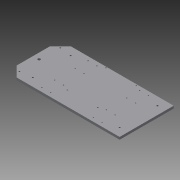
# Autodesk Inventor part: BaseNEW
Saved by Autodesk Inventor 2015 (Build 190159000, 159)
## iProperties
Created: 2015-04-03
Part Number: BaseNEW
Material: Generic
Document SubType Name: Modeling
Designer: Judson
Density: 1 g/cm^3
Appearance: Default
Author: Judson
Autodesk Inventor part; units mm, degrees
ref_plane "YZ Plane" through (0, 0, 0) normal (1, 0, 0) x (0, 1, 0)
ref_plane "XZ Plane" through (0, 0, 0) normal (0, 1, 0) x (-1, 0, 0)
ref_plane "XY Plane" through (0, 0, 0) normal (0, 0, 1) x (1, 0, 0)
sketch "Sketch1" plane through (0, 0, 0) normal (0, 1, 0) x (-1, 0, 0)
  line L0 (139.7, 66.675) -> (-139.7, 66.675)
  line L1 (-139.7, 66.675) -> (-139.7, -66.675)
  line L2 (-139.7, -66.675) -> (139.7, -66.675)
  line L3 (139.7, -66.675) -> (139.7, 66.675)
  line L4 (114.3, 66.675) -> (114.3, -66.675)
  line L5 (114.3, 66.675) -> (139.7, 41.275)
  line L6 (114.3, -66.675) -> (139.7, -41.275)
  point P0 (0, 0)
  dimension "d0" = 133.35
  dimension "d1" = 279.4
  dimension "d2" = 66.675
  dimension "d3" = 139.7
  dimension "d4" = 25.4
  dimension "d5" = 45
  dimension "d6" = 45
  constraints: 14 end point, 4 point on line, 2 parallel, 2 perpendicular, 1 horizontal
  measures "d0" distance of L0.end L1.end
  measures "d1" distance of L1.end L2.end
  measures "d2" distance from line of point (0, 0) L2
  measures "d3" distance from line of point (0, 0) L1
  measures "d4" distance between parallel lines of L4 L3
  measures "d5" angle of L2 L6
  measures "d6" angle of L4 L5
extrude "Body" add sketch "Sketch1" along normal blind 5.9944 contours L4 L2 L1 L0 | L5 L3 L6 L4
sketch "Sketch2" plane through (0, 5.9944, 0) normal (0, 1, 0) x (1, 0, 0)
  line L0 (-114.3, 66.675) -> (-139.7, 41.275) projected
  line L1 (-139.7, 41.275) -> (-139.7, -41.275) projected
  line L2 (-139.7, -41.275) -> (-114.3, -66.675) projected
  line L3 (-114.3, -66.675) -> (139.7, -66.675) projected
  line L4 (139.7, -66.675) -> (139.7, 66.675) projected
  line L5 (139.7, 66.675) -> (-114.3, 66.675) projected
  line L6 (-114.3, -66.675) -> (-114.3, 66.675)
  line L7 (-114.3, -14.605) -> (139.7, -14.605)
  line L8 (76.2, -14.605) -> (76.2, -66.675)
  line L9 (-50.8, -14.605) -> (-50.8, -66.675)
  line L10 (-114.3, -66.675) -> (139.7, -66.675) projected
  line L11 (-40.005, -14.605) -> (-40.005, -66.675)
  line L12 (-40.005, -66.675) -> (-61.595, -66.675)
  line L13 (-61.595, -66.675) -> (-61.595, -14.605)
  line L14 (12.7, -66.675) -> (12.7, 66.675)
  line L15 (76.2, -14.605) -> (76.2, -66.675)
  line L16 (65.405, -14.605) -> (65.405, -66.675)
  line L17 (86.995, -66.675) -> (86.995, -14.605)
  circle A0 centre (-61.595, -57.023) radius 1.27
  circle A1 centre (-61.595, -25.273) radius 1.27
  circle A2 centre (-40.005, -57.023) radius 1.27
  circle A3 centre (-40.005, -25.273) radius 1.27
  circle A4 centre (86.995, -57.023) radius 1.27
  circle A5 centre (86.995, -25.273) radius 1.27
  circle A6 centre (65.405, -25.273) radius 1.27
  circle A7 centre (65.405, -57.023) radius 1.27
  line L18 (-139.7, 0) -> (139.7, 0)
  line L19 (-114.3, 14.605) -> (139.7, 14.605)
  line L20 (76.2, 14.605) -> (76.2, 66.675)
  line L21 (-50.8, 14.605) -> (-50.8, 66.675)
  line L22 (-40.005, 14.605) -> (-40.005, 66.675)
  line L23 (-61.595, 66.675) -> (-61.595, 14.605)
  line L24 (65.405, 14.605) -> (65.405, 66.675)
  line L25 (86.995, 66.675) -> (86.995, 14.605)
  circle A8 centre (-61.595, 57.023) radius 1.27
  circle A9 centre (-61.595, 25.273) radius 1.27
  circle A10 centre (-40.005, 25.273) radius 1.27
  circle A11 centre (-40.005, 57.023) radius 1.27
  circle A12 centre (86.995, 25.273) radius 1.27
  circle A13 centre (65.405, 25.273) radius 1.27
  circle A14 centre (65.405, 57.023) radius 1.27
  circle A15 centre (86.995, 57.023) radius 1.27
  point P0 (0, 0)
  dimension "d10" = 52.07
  dimension "d11" = 63.5
  dimension "d12" = 63.5
  dimension "d13" = 21.59
  dimension "d14" = 10.795
  dimension "d15" = 127
  dimension "d16" = 2.54
  dimension "d17" = 9.652
  dimension "d18" = 2.54
  dimension "d19" = 10.668
  constraints: 38 end point, 32 symmetric about line, 17 point on line, 16 centre point, 4 midpoint, 4 perpendicular, 1 parallel, 1 vertical, 14 other
  measures "d10" distance between parallel lines of L3 L7
  measures "d11" distance between parallel lines of L4 L8
  measures "d12" distance between parallel lines of L6 L9
  measures "d13" distance between parallel lines of L13 L11
  measures "d14" distance between parallel lines of L9 L11
  measures "d15" distance between parallel lines of L6 L14
  measures "d16" diameter of A0
  measures "d17" distance from line of L3 A0.centre
  measures "d18" diameter of A1
  measures "d19" distance from line of L7 A1.centre
extrude "Motor Mounts" cut sketch "Sketch2" against normal blind 5.9944 contours A8 L23 | L23 A8 | A9 L23 | L23 A9 | A11 L22 | L22 A11 | A10 L22 | L22 A10 | A1 L13 | L13 A1 | A0 L13 | L13 A0 | A14 L24 | L24 A14 | A3 L11 | L11 A3 | A6 L16 | L16 A6 | A13 L24 | L24 A13 | A2 L11 | L11 A2 | A7 L16 | L16 A7 | A5 L17 | L17 A5 | A12 L25 | L25 A12 | A15 L25 | L25 A15 | A4 L17 | L17 A4
sketch "Sketch3" plane through (0, 5.9944, 0) normal (0, 1, 0) x (1, 0, 0)
  circle A0 centre (65.405, 57.023) radius 1.27 projected
  circle A1 centre (65.405, 25.273) radius 1.27 projected
  circle A2 centre (-61.595, 57.023) radius 1.27 projected
  circle A3 centre (-61.595, 25.273) radius 1.27 projected
  circle A4 centre (-61.595, -25.273) radius 1.27 projected
  circle A5 centre (-40.005, -57.023) radius 1.27 projected
  circle A6 centre (65.405, -57.023) radius 1.27 projected
  circle A7 centre (86.995, -57.023) radius 1.27 projected
  circle A8 centre (86.995, -25.273) radius 1.27 projected
  circle A9 centre (65.405, -25.273) radius 1.27 projected
  circle A10 centre (-40.005, -25.273) radius 1.27 projected
  circle A11 centre (-61.595, -57.023) radius 1.27 projected
  circle A12 centre (-40.005, 25.273) radius 1.27 projected
  circle A13 centre (-40.005, 57.023) radius 1.27 projected
  circle A14 centre (86.995, 25.273) radius 1.27 projected
  circle A15 centre (86.995, 57.023) radius 1.27 projected
  line L0 (-114.3, 66.675) -> (-139.7, 41.275) projected
  line L1 (-139.7, 41.275) -> (-139.7, -41.275) projected
  line L2 (-139.7, -41.275) -> (-114.3, -66.675) projected
  line L3 (-114.3, -66.675) -> (139.7, -66.675) projected
  line L4 (139.7, -66.675) -> (139.7, 66.675) projected
  line L5 (139.7, 66.675) -> (-114.3, 66.675) projected
  line L6 (-139.7, 0) -> (139.7, 0)
  line L7 (-114.3, 66.675) -> (-114.3, -66.675)
  line L8 (139.7, 66.675) -> (-114.3, 66.675) projected
  line L9 (12.7, 66.675) -> (12.7, -66.675)
  line L10 (52.7, 66.675) -> (-27.3, 66.675)
  circle A16 centre (50.16, 64.135) radius 1.397
  line L11 (-27.3, 66.675) -> (52.7, 66.675)
  line L12 (52.7, 66.675) -> (52.7, -33.325)
  line L13 (52.7, -33.325) -> (-27.3, -33.325)
  line L14 (-27.3, -33.325) -> (-27.3, 66.675)
  circle A17 centre (-24.76, 64.135) radius 1.397
  line L15 (52.7, 16.675) -> (-27.3, 16.675)
  circle A18 centre (50.16, -30.785) radius 1.397
  circle A19 centre (-24.76, -30.785) radius 1.397
  point P0 (0, 0)
  point P1 (12.7, 0)
  dimension "d22" = 127
  dimension "d25" = 2.54
  dimension "d27" = 2.794
  dimension "d50" = 2.54
  dimension "d51" = 100
  dimension "d52" = 80
  dimension "d53" = 40
  dimension "d54" = 40
  dimension "d55" = 2.54
  dimension "d56" = 50
  constraints: 18 end point, 7 midpoint, 4 centre point, 4 perpendicular, 3 symmetric about line, 2 horizontal, 2 parallel, 3 other
  measures "d22" distance between parallel lines of L4 L9
  measures "d25" distance from line of L10 A16.centre
  measures "d27" diameter of A16
  measures "d50" distance from line of L5 A16.centre
  measures "d51" distance of L11.end L12.end
  measures "d52" distance of L12.end L13.end
  measures "d53" distance between parallel lines of L9 L12
  measures "d54" distance between parallel lines of L14 L9
  measures "d55" distance from line of L12 A16.centre
  measures "d56" distance between parallel lines of L5 L15
extrude "PCB Mounts" cut sketch "Sketch3" against normal blind 5.9944 contours A16 | A17 | A18 | A19
sketch "Sketch4" plane through (0, 5.9944, 0) normal (0, 1, 0) x (1, 0, 0)
  circle A0 centre (65.405, 57.023) radius 1.27 projected
  circle A1 centre (65.405, 25.273) radius 1.27 projected
  circle A2 centre (-61.595, 57.023) radius 1.27 projected
  circle A3 centre (-61.595, 25.273) radius 1.27 projected
  circle A4 centre (-61.595, -25.273) radius 1.27 projected
  circle A5 centre (-40.005, -57.023) radius 1.27 projected
  circle A6 centre (65.405, -57.023) radius 1.27 projected
  circle A7 centre (86.995, -57.023) radius 1.27 projected
  circle A8 centre (86.995, -25.273) radius 1.27 projected
  circle A9 centre (65.405, -25.273) radius 1.27 projected
  circle A10 centre (-40.005, -25.273) radius 1.27 projected
  circle A11 centre (-61.595, -57.023) radius 1.27 projected
  circle A12 centre (-40.005, 25.273) radius 1.27 projected
  circle A13 centre (-40.005, 57.023) radius 1.27 projected
  circle A14 centre (86.995, 25.273) radius 1.27 projected
  circle A15 centre (86.995, 57.023) radius 1.27 projected
  line L0 (-114.3, 66.675) -> (-139.7, 41.275) projected
  line L1 (-139.7, 41.275) -> (-139.7, -41.275) projected
  line L2 (-139.7, -41.275) -> (-114.3, -66.675) projected
  line L3 (-114.3, -66.675) -> (139.7, -66.675) projected
  line L4 (139.7, -66.675) -> (139.7, 66.675) projected
  line L5 (139.7, 66.675) -> (-114.3, 66.675) projected
  line L6 (-114.3, 66.675) -> (-114.3, -66.675)
  line L7 (-139.7, 0) -> (-114.3, 0)
  circle A16 centre (-125.385, 0) radius 3.205
  point P0 (0, 0)
  dimension "d30" = 14.315
  dimension "d31" = 6.41
  constraints: 4 end point, 2 midpoint, 1 centre point, 1 vertical
  measures "d30" distance from line of L1 A16.centre
  measures "d31" diameter of A16
extrude "ARLO Mount" cut sketch "Sketch4" against normal blind 25.4 contours A16 L7 | L7 A16
sketch "Sketch5" plane through (0, 5.9944, 0) normal (0, 1, 0) x (1, 0, 0)
  circle A0 centre (-125.385, 0) radius 3.205 projected
  circle A1 centre (65.405, 57.023) radius 1.27 projected
  circle A2 centre (65.405, 25.273) radius 1.27 projected
  circle A3 centre (-61.595, 57.023) radius 1.27 projected
  circle A4 centre (-61.595, 25.273) radius 1.27 projected
  circle A5 centre (-61.595, -25.273) radius 1.27 projected
  circle A6 centre (-40.005, -57.023) radius 1.27 projected
  circle A7 centre (65.405, -57.023) radius 1.27 projected
  circle A8 centre (86.995, -57.023) radius 1.27 projected
  circle A9 centre (86.995, -25.273) radius 1.27 projected
  circle A10 centre (65.405, -25.273) radius 1.27 projected
  circle A11 centre (-40.005, -25.273) radius 1.27 projected
  circle A12 centre (-61.595, -57.023) radius 1.27 projected
  circle A13 centre (-40.005, 25.273) radius 1.27 projected
  circle A14 centre (-40.005, 57.023) radius 1.27 projected
  circle A15 centre (86.995, 25.273) radius 1.27 projected
  circle A16 centre (86.995, 57.023) radius 1.27 projected
  line L0 (139.7, 66.675) -> (139.7, -66.675) projected
  line L1 (139.7, -66.675) -> (-114.3, -66.675) projected
  line L2 (-114.3, -66.675) -> (-139.7, -41.275) projected
  line L3 (-139.7, -41.275) -> (-139.7, 41.275) projected
  line L4 (-139.7, 41.275) -> (-114.3, 66.675) projected
  line L5 (-114.3, 66.675) -> (139.7, 66.675) projected
  line L6 (-114.3, 66.675) -> (-114.3, -66.675)
  line L7 (-139.7, 41.275) -> (-136.1645, 37.7395)
  line L8 (-114.3, -66.675) -> (-110.7645, -63.1395)
  line L9 (-139.7, -41.275) -> (-114.3, -66.675)
  line L10 (-136.1645, -37.7395) -> (-110.7645, -63.1395)
  circle A17 centre (-123.4645, -50.4395) radius 1.651
  line L11 (-114.3, 66.675) -> (-139.7, 41.275)
  line L12 (-136.1645, 37.7395) -> (-110.7645, 63.1395)
  circle A18 centre (-123.4645, 50.4395) radius 1.651
  line L13 (-114.3, 66.675) -> (-110.7645, 63.1395)
  line L14 (-139.7, -41.275) -> (-136.1645, -37.7395)
  circle A19 centre (50.16, 64.135) radius 1.397 projected
  circle A20 centre (50.16, -30.785) radius 1.397 projected
  circle A21 centre (-24.76, -30.785) radius 1.397 projected
  circle A22 centre (-24.76, 64.135) radius 1.397 projected
  point P0 (0, 0)
  dimension "d36" = 5
  dimension "d37" = 17.9605
  dimension "d38" = 5
  dimension "d39" = 3.302
  dimension "d40" = 3.302
  dimension "d41" = 17.9605
  constraints: 18 end point, 3 perpendicular, 2 centre point, 2 midpoint, 1 vertical
  measures "d36" distance between parallel lines of L2 L10
  measures "d37" distance from line of L8 A17.centre
  measures "d38" distance between parallel lines of L4 L12
  measures "d39" diameter of A18
  measures "d40" diameter of A17
  measures "d41" distance from line of L7 A18.centre
extrude "IR Mounts" cut sketch "Sketch5" against normal blind 25.4 contours A18 L12 | L12 A18 | A17 L10 | L10 A17
sketch "Sketch6" plane through (0, 5.9944, 0) normal (0, 1, 0) x (1, 0, 0)
  circle A0 centre (-123.4645, 50.4395) radius 1.651 projected
  circle A1 centre (-123.4645, -50.4395) radius 1.651 projected
  circle A2 centre (-125.385, 0) radius 3.205 projected
  circle A3 centre (65.405, 57.023) radius 1.27 projected
  circle A4 centre (65.405, 25.273) radius 1.27 projected
  circle A5 centre (-61.595, 57.023) radius 1.27 projected
  circle A6 centre (-61.595, 25.273) radius 1.27 projected
  circle A7 centre (-61.595, -25.273) radius 1.27 projected
  circle A8 centre (-40.005, -57.023) radius 1.27 projected
  circle A9 centre (65.405, -57.023) radius 1.27 projected
  circle A10 centre (86.995, -57.023) radius 1.27 projected
  circle A11 centre (86.995, -25.273) radius 1.27 projected
  circle A12 centre (65.405, -25.273) radius 1.27 projected
  circle A13 centre (-40.005, -25.273) radius 1.27 projected
  circle A14 centre (-61.595, -57.023) radius 1.27 projected
  circle A15 centre (-40.005, 25.273) radius 1.27 projected
  circle A16 centre (-40.005, 57.023) radius 1.27 projected
  circle A17 centre (86.995, 25.273) radius 1.27 projected
  circle A18 centre (86.995, 57.023) radius 1.27 projected
  line L0 (139.7, 66.675) -> (139.7, -66.675) projected
  line L1 (139.7, -66.675) -> (-114.3, -66.675) projected
  line L2 (-114.3, -66.675) -> (-139.7, -41.275) projected
  line L3 (-139.7, -41.275) -> (-139.7, 41.275) projected
  line L4 (-139.7, 41.275) -> (-114.3, 66.675) projected
  line L5 (-114.3, 66.675) -> (139.7, 66.675) projected
  line L6 (-114.3, 66.675) -> (-114.3, -66.675)
  line L7 (12.7, 66.675) -> (12.7, -66.675)
  line L8 (-114.3, 0) -> (139.7, 0)
  line L9 (139.7, -66.675) -> (139.7, 66.675) projected
  circle A19 centre (-94.3, 46.675) radius 1.905
  circle A20 centre (-94.3, -46.675) radius 1.905
  circle A21 centre (119.7, 46.675) radius 1.905
  circle A22 centre (119.7, -46.675) radius 1.905
  circle A23 centre (50.16, 64.135) radius 1.397 projected
  circle A24 centre (50.16, -30.785) radius 1.397 projected
  circle A25 centre (-24.76, -30.785) radius 1.397 projected
  circle A26 centre (-24.76, 64.135) radius 1.397 projected
  point P0 (0, 0)
  dimension "d44" = 127
  dimension "d45" = 3.81
  dimension "d46" = 20
  dimension "d47" = 20
  constraints: 6 end point, 4 centre point, 4 midpoint, 3 symmetric about line, 1 perpendicular, 3 other
  measures "d44" distance between parallel lines of L6 L7
  measures "d45" diameter of A19
  measures "d46" horizontal distance of A19.centre L4.end
  measures "d47" distance from line of L5 A19.centre
extrude "Standoff Mounts" cut sketch "Sketch6" against normal blind 25.4 contours A19 | A20 | A21 | A22
body "Solid1"
